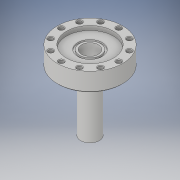
# Autodesk Inventor part: universal connector
Saved by Autodesk Inventor 2018 (Build 220112000, 112)
## iProperties
Created: 2019-01-21
Part Number: universal connector
Material: Generic
Document SubType Name: Modeling
Designer: Admin
Density: 1 g/cm^3
Appearance: Default
Author: Admin
Autodesk Inventor part; units mm, degrees
ref_plane "YZ Plane" through (0, 0, 0) normal (1, 0, 0) x (0, 1, 0)
ref_plane "XZ Plane" through (0, 0, 0) normal (0, 1, 0) x (-1, 0, 0)
ref_plane "XY Plane" through (0, 0, 0) normal (0, 0, 1) x (1, 0, 0)
sketch "Sketch1" plane through (0, 0, 0) normal (0, 1, 0) x (-1, 0, 0)
  circle A0 centre (0, 0) radius 22.2885
  dimension "d0" = 44.577
  constraints: 1 centre point, 1 coincident
  measures "d0" diameter of A0
extrude "Extrusion1" add sketch "Sketch1" along normal blind 12.7
chamfer "Chamfer1" distance 0.7384 angle 45 1 edges at (22.2885, 0, 0)
sketch "Sketch2" plane through (0, 12.7, 0) normal (0, 1, 0) x (1, 0, 0)
  circle A0 centre (0, 0) radius 16.002
  dimension "d6" = 32.004
  constraints: 1 centre point, 1 coincident
  measures "d6" diameter of A0
extrude "Extrusion2" cut sketch "Sketch2" against normal blind 2.8702
sketch "Sketch3" plane through (0, 9.8298, 0) normal (0, 1, 0) x (1, 0, 0)
  circle A0 centre (0, 0) radius 8.3566
  circle A1 centre (0, 0) radius 7.0866
  dimension "d9" = 16.7132
  dimension "d10" = 1.27
  constraints: 2 centre point, 2 coincident
  measures "d9" diameter of A0
  measures "d10" radial gap between concentric circles of A1 A0
extrude "Extrusion3" cut sketch "Sketch3" against normal blind 1.016
sketch "Sketch4" plane through (0, 9.8298, 0) normal (0, 1, 0) x (1, 0, 0)
  circle A0 centre (0, 0) radius 6.35
  dimension "d13" = 12.7
  constraints: 1 centre point, 1 coincident
  measures "d13" diameter of A0
extrude "Extrusion4" cut sketch "Sketch4" against normal up to surface (9.8298 mm away)
chamfer "Chamfer2" distance 0.7384 angle 45 1 edges at (-6.35, 0, 0)
sketch "Sketch5" plane through (0, 9.8298, 0) normal (0, 1, 0) x (1, 0, 0)
  circle A0 centre (0, 0) radius 6.35
  circle A1 centre (0, 0) radius 5.715
  circle A2 centre (0, 0) radius 6.35 projected
  dimension "d19" = 11.43
  constraints: 2 centre point, 2 coincident, 1 concentric
  measures "d19" diameter of A1
extrude "Extrusion5" add sketch "Sketch5" against normal blind 50.8
sketch "Sketch6" plane through (0, 12.7, 0) normal (0, 1, 0) x (1, 0, 0)
  line L0 (0, 0) -> (17.0477, 9.8425) construction
  line L1 (0, 0) -> (19.685, 0) construction
  dimension "d22" = 19.685
  dimension "d23" = 30
  constraints: 4 end point, 1 coincident, 1 equal length, 1 horizontal
  measures "d22" distance of L0.start L0.end
  measures "d23" angle of L1 L0
hole "Hole1" at (17.0477, 12.7, -9.8425) direction (0, -1, 0) diameter 3.175 end through all
chamfer "Chamfer3" distance 0.381 angle 45 1 edges at (17.0477, 12.7, -11.43)
pattern_circular "Circular Pattern1" count 12 over 360 about axis through (0, 9.8298, 0) along (0, -1, 0) of "Hole1", "Chamfer3"
body "Solid1"
